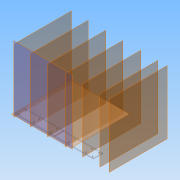
# Autodesk Inventor part: Pancake_Catch Backboard_4 Lanes
Saved by Autodesk Inventor 2018.1 (Build 221171000, 171)
## iProperties
Created: 2019-02-21
Part Number: Pancake_Catch Backboard_4 Lanes
Material: PET Plastic
Document SubType Name: Modeling
Designer: James
Density: 1.541 g/cm^3
Appearance: Polycarbonate - Clear
Author: James
Autodesk Inventor part; units mm, degrees
ref_plane "YZ Plane" through (0, 0, 0) normal (1, 0, 0) x (0, 1, 0)
ref_plane "XZ Plane" through (0, 0, 0) normal (0, 1, 0) x (-1, 0, 0)
ref_plane "XY Plane" through (0, 0, 0) normal (0, 0, 1) x (1, 0, 0)
derived "Pancake_Skeleton.ipt"
ref_plane "Ground" through (0, 0, 0) normal (0, 1, 0) x (-1, 0, 0)
ref_plane "Back" through (0, 0, 0) normal (0, 0, 1) x (1, 0, 0)
ref_plane "LHS" through (0, 0, 0) normal (1, 0, 0) x (0, 1, 0)
ref_plane "Lane 1" through (90, 0, 0) normal (1, 0, 0) x (0, 1, 0)
ref_plane "Lane 2" through (185, 0, 0) normal (1, 0, 0) x (0, 1, 0)
ref_plane "Lane 3" through (280, 0, 0) normal (1, 0, 0) x (0, 1, 0)
ref_plane "Lane 4" through (375, 0, 0) normal (1, 0, 0) x (0, 1, 0)
ref_plane "Lane 5" through (470, 0, 0) normal (1, 0, 0) x (0, 1, 0)
ref_plane "RHS" through (520, 0, 0) normal (1, 0, 0) x (0, 1, 0)
sketch "Sketch1" plane through (0, 0, 0) normal (0, 0, 1) x (1, 0, 0)
  line L0 (0, 60) -> (0, -10) projected
  line L1 (-85, 0) -> (510, 0) projected
  line L2 (0, 0) -> (425, 0)
  line L3 (425, 0) -> (425, 50)
  line L4 (425, 50) -> (0, 50)
  line L5 (0, 50) -> (0, 0)
  line L6 (520, 60) -> (520, -10) projected
  dimension "d1" = 50
  dimension "d28" = 95
  constraints: 8 end point, 2 parallel, 1 horizontal, 1 perpendicular
  measures "d1" distance of L2.end L3.end
  measures "d28" distance between parallel lines of L6 L3
extrude "Extrusion1" add sketch "Sketch1" along normal blind 5
sketch "Sketch2" plane through (0, 0, 5) normal (0, 0, 1) x (1, 0, 0)
  line L0 (90, 60) -> (90, -10) projected
  line L1 (-85, 0) -> (510, 0) projected
  line L2 (425, 50) -> (0, 50) projected
  point P0 (0, 0)
  point P1 (90, 10)
  point P2 (90, 40)
  dimension "d4" = 30
  dimension "d5" = 10
  dimension "d6" = 10
  constraints: 1 point on line, 1 vertical alignment
  measures "d4" distance of point (90, 40) point (90, 10)
  measures "d5" distance from line of L1 point (90, 10)
  measures "d6" distance from line of L2 point (90, 40)
hole "Hole1" at (90, 10, 5) at (90, 40, 5) direction (0, 0, -1) diameter 4.5 end through all clearance for "Socket Head Cap Screw" size "M4" standard "Ansi Metric M Profile"
pattern_linear "Rectangular Pattern1" count 4 spacing 95 along (1, 0, 0) of "Hole1"
sketch "Sketch3" plane through (0, 0, 5) normal (0, 0, 1) x (1, 0, 0)
  line L0 (0, 60) -> (0, -10) projected
  line L1 (425, 50) -> (0, 50) projected
  line L2 (-104, 0) -> (624, 0) projected
  point P0 (0, 0)
  point P1 (12.5, 42.5)
  point P2 (12.5, 7.5)
  dimension "d17" = 12.5
  dimension "d18" = 35
  dimension "d19" = 7.5
  dimension "d20" = 7.5
  constraints: 1 vertical alignment
  measures "d17" distance from line of point (12.5, 42.5) L0
  measures "d18" distance of point (12.5, 7.5) point (12.5, 42.5)
  measures "d19" distance from line of L1 point (12.5, 42.5)
  measures "d20" distance from line of L2 point (12.5, 7.5)
hole "Hole2" at (12.5, 42.5, 5) at (12.5, 7.5, 5) direction (0, 0, -1) diameter 4.5 end through all clearance for "Socket Head Cap Screw" size "M4" standard "Ansi Metric M Profile"
ref_plane "Mid Plane" through (212.5, 0, 0) normal (-1, 0, 0) x (0, 0, 1)
mirror "Mirror1" about plane through (212.5, 0, 0) normal (-1, 0, 0) of "Hole2"
equation "\"d5\" = d6"
equation "\"d19\" = d20"
body "Solid1"
